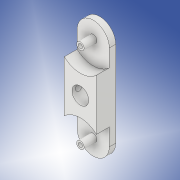
# Autodesk Inventor part: WaveGenerator
Saved by Autodesk Inventor 2017 SP1 (Build 210196100, 196)
## iProperties
Created: 2017-07-11
Part Number: WaveGenerator
Material: ABS Plastic
Document SubType Name: Modeling
Designer: zallen
Density: 1.06 g/cm^3
Appearance: CR White
Author: zallen
Autodesk Inventor part; units mm, degrees
ref_plane "YZ Plane" through (0, 0, 0) normal (1, 0, 0) x (0, 1, 0)
ref_plane "XZ Plane" through (0, 0, 0) normal (0, 1, 0) x (-1, 0, 0)
ref_plane "XY Plane" through (0, 0, 0) normal (0, 0, 1) x (1, 0, 0)
sketch "Sketch1" plane through (0, 0, 0) normal (0, 0, 1) x (1, 0, 0)
  line L0 (0, 0) -> (0, 55) construction
  circle A0 centre (0, 47.5) radius 7.5 construction
  circle A1 centre (0, 7.5) radius 7.5 construction
  line L1 (7.5, 47.5) -> (7.5, 7.5)
  line L2 (-7.5, 7.5) -> (-7.5, 47.5)
  arc A2 (7.5, 47.5) -> (-7.5, 47.5) centre (0, 47.5) ccw
  arc A3 (-7.5, 7.5) -> (7.5, 7.5) centre (0, 7.5) ccw
  circle A4 centre (0, 27.5) radius 3.9
  circle A5 centre (0, 47.5) radius 1.75
  circle A6 centre (0, 7.5) radius 1.75
  dimension "d1" = 15
  dimension "d2" = 15
  dimension "d3" = 7.8
  dimension "d4" = 3.5
  dimension "d5" = 3.5
  dimension "d21" = 40
  constraints: 10 point on circle, 7 centre point, 6 end point, 6 tangent, 2 coincident, 2 point on line, 1 concentric, 1 midpoint, 1 vertical
  measures "d1" diameter of A0
  measures "d2" diameter of A1
  measures "d3" diameter of A4
  measures "d4" diameter of A5
  measures "d5" diameter of A6
  measures "d21" distance of A0.centre A1.centre
extrude "Extrusion1" add sketch "Sketch1" along normal blind 3
sketch "Sketch3" plane through (0, 0, 0) normal (0, 0, -1) x (-1, 0, 0)
  circle A0 centre (0, 47.5) radius 1.75 projected
  circle A1 centre (0, 7.5) radius 1.75 projected
  point P0 (0, 0)
extrude "Extrusion2" add sketch "Sketch3" against normal blind 9
sketch "Sketch4" plane through (0, 47.5, 9) normal (0, 0, 1) x (1, 0, 0)
  circle A0 centre (0, 0) radius 1.75 projected
  circle A1 centre (0, -40) radius 1.75 projected
  circle A2 centre (0, 0) radius 1
  circle A3 centre (0, -40) radius 1
  point P0 (0, -47.5)
  dimension "d10" = 2
  dimension "d11" = 2
  constraints: 2 centre point, 2 coincident
  measures "d10" diameter of A2
  measures "d11" diameter of A3
extrude "Extrusion3" cut sketch "Sketch4" against normal through all contours A2 | A3
sketch "Sketch5" plane through (0, 0, 3) normal (0, 0, 1) x (1, 0, 0)
  arc A0 (7.5, 47.5) -> (-7.5, 47.5) centre (0, 47.5) ccw projected
  arc A1 (-7.5, 7.5) -> (7.5, 7.5) centre (0, 7.5) ccw projected
  circle A2 centre (0, 47.5) radius 1 projected
  circle A3 centre (0, 47.5) radius 11 construction
  circle A4 centre (0, 7.5) radius 11 construction
  line L0 (7.5, 7.5) -> (7.5, 47.5) projected
  line L1 (7.5, 39.4533) -> (7.5, 15.5467)
  line L2 (-7.5, 47.5) -> (-7.5, 7.5) projected
  line L3 (-7.5, 39.4533) -> (-7.5, 15.5467)
  arc A5 (-7.5, 39.4533) -> (7.5, 39.4533) centre (0, 47.5) ccw
  arc A6 (7.5, 15.5467) -> (-7.5, 15.5467) centre (0, 7.5) ccw
  circle A7 centre (0, 27.5) radius 3.9 projected
  point P0 (0, 0)
  dimension "d14" = 22
  dimension "d15" = 22
  constraints: 8 point on circle, 4 centre point, 4 end point, 4 point on line, 2 coincident, 2 concentric
  measures "d14" diameter of A3
  measures "d15" diameter of A4
extrude "Extrusion4" add sketch "Sketch5" along normal blind 6 contours L0 A6 L2 A5
sketch "Sketch6" plane through (0, 0, 0) normal (1, 0, 0) x (0, 1, 0)
  line L0 (7.5, 0) -> (47.5, 0) projected
  line L1 (7.5, 0) -> (7.5, 3) projected
  line L2 (15.5467, 3) -> (7.5, 3) projected
  line L3 (15.5467, 3) -> (15.5467, 9) projected
  line L4 (39.4533, 9) -> (15.5467, 9) projected
  line L5 (39.4533, 3) -> (39.4533, 9) projected
  line L6 (47.5, 0) -> (47.5, 3) projected
  circle A0 centre (27.5, 6) radius 1.5
  line L7 (47.5, 3) -> (39.4533, 3) projected
  point P0 (0, 0)
  point P1 (27.5, 9)
  point P2 (39.4533, 6)
  dimension "d18" = 3
  constraints: 2 midpoint, 1 centre point, 1 horizontal alignment, 1 vertical alignment
  measures "d18" diameter of A0
extrude "Extrusion5" cut sketch "Sketch6" against normal through all contours A0
equation "\"d5\" = d4"
equation "\"d15\" = d14"
body "Solid1"
